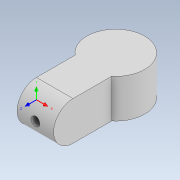
# Autodesk Inventor part: thigh_inventor
Saved by Autodesk Inventor 2020 (Build 240168000, 168)
## iProperties
Created: 2021-01-07
Part Number: thigh_inventor
Material: Generic
Document SubType Name: Modeling
Designer: DELL
Density: 1 g/cm^3
Appearance: Default
Author: DELL
Autodesk Inventor part; units mm, degrees
ref_plane "YZ Plane" through (0, 0, 0) normal (1, 0, 0) x (0, 1, 0)
ref_plane "XZ Plane" through (0, 0, 0) normal (0, 1, 0) x (-1, 0, 0)
sketch "Sketch1" plane through (0, 0, 0) normal (0, 1, 0) x (-1, 0, 0)
  line L0 (0, 0) -> (-50, 0)
  line L1 (-50, 0) -> (-50, -83.5)
  line L2 (-50, -83.5) -> (0, -83.5)
  line L3 (0, -83.5) -> (0, 0)
  circle A0 centre (-25, -83.5) radius 39.5
  point P0 (-50, -52.9181)
  point P1 (0, -52.9181)
  dimension "d0" = 50
  dimension "d1" = 79
  dimension "d14" = 83.5
  constraints: 8 end point, 2 parallel, 1 centre point, 1 horizontal, 1 midpoint, 1 perpendicular
  measures "d0" distance between parallel lines of L1 L3
  measures "d1" diameter of A0
  measures "d14" distance between parallel lines of L0 L2
extrude "Extrusion1" add sketch "Sketch1" along normal mid plane 53
sketch "Sketch2" plane through (0, 0, 0) normal (1, 0, 0) x (0, 1, 0)
  line L0 (26.5, 0) -> (-26.5, 0) projected
  circle A0 centre (0, 0) radius 26.5
  constraints: 1 midpoint, 3 other
extrude "Extrusion2" add sketch "Sketch2" along normal up to surface (50 mm away) contours L0 A0 picked at (8.0782, 6.219)
ref_plane "Work Plane1" through (25, 0, -44) normal (0, 0, 1) x (1, 0, 0)
sketch "Sketch3" plane through (25, 0, -44) normal (0, 0, 1) x (1, 0, 0)
  circle A0 centre (0, 0) radius 6
  line L0 (-25, 0) -> (27.9863, 0) construction
  line L1 (39.5, 26.5) -> (-39.5, 26.5) construction
  line L2 (0, 26.5) -> (0, -26.5) construction
  point P0 (25, 26.5)
  point P1 (-25, 26.5)
  dimension "d15" = 12
  constraints: 4 end point, 2 midpoint, 1 centre point, 1 coincident, 1 horizontal, 1 point on line, 1 vertical
  measures "d15" diameter of A0
extrude "Extrusion3" cut sketch "Sketch3" along normal through all
body "Solid1"
